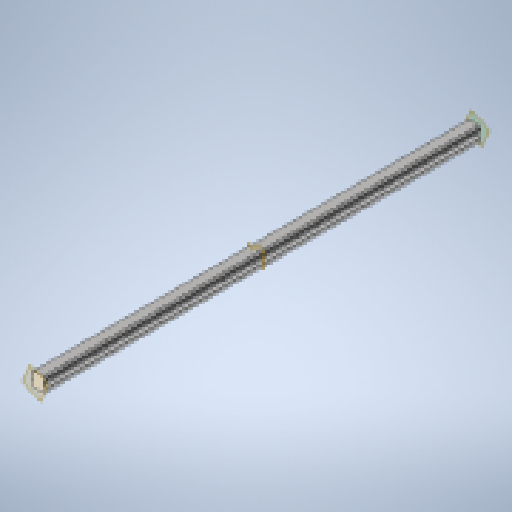
# Autodesk Inventor part: HGR15_Y_RAIL
Saved by Autodesk Inventor 2025.2 (Build 292293000, 293)
## iProperties
Created: 2026-02-05
Part Number: HGR15_Y_RAIL
Material: Generic
Document SubType Name: Modeling
Designer: composite
Density: 1 g/cm^3
Appearance: Default
Author: composite
Autodesk Inventor part; units mm, degrees
ref_plane "YZ Plane" through (0, 0, 0) normal (1, 0, 0) x (0, 1, 0)
ref_plane "XZ Plane" through (0, 0, 0) normal (0, 1, 0) x (-1, 0, 0)
ref_plane "XY Plane" through (0, 0, 0) normal (0, 0, 1) x (1, 0, 0)
derived "HGR15_REPRESENTATIVE.ipt"
sketch "hgr15 REP SKETCH" plane through (-6.8, 0, 100) normal (0, 0, 1) x (1, 0, 0)
  arc A0 (-0.4071, 3.9505) -> (-0.7, 3.2434) centre (0.3, 3.2434) ccw
  line L0 (-0.7, 3.2434) -> (-0.7, 0.7)
  line L1 (-0.7, 0.7) -> (0, 0)
  line L2 (0, 0) -> (13.6, 0)
  line L3 (13.6, 0) -> (14.3, 0.7)
  line L4 (14.3, 0.7) -> (14.3, 3.2434)
  arc A1 (14.3, 3.2434) -> (14.0071, 3.9505) centre (13.3, 3.2434) ccw
  line L5 (14.0071, 3.9505) -> (11.6872, 6.2704)
  arc A2 (11.57, 6.5533) -> (11.6872, 6.2704) centre (11.97, 6.5533) ccw
  line L6 (11.57, 6.5533) -> (11.57, 8.1153)
  arc A3 (11.6872, 8.3982) -> (11.57, 8.1153) centre (11.97, 8.1153) ccw
  line L7 (11.6872, 8.3982) -> (11.8816, 8.5926)
  arc A4 (11.8816, 8.5926) -> (12.0706, 9.0718) centre (11.6914, 8.9445) ccw
  arc A5 (13.2785, 10.4123) -> (12.0706, 9.0718) centre (13.6562, 8.8576) ccw
  arc A6 (13.2785, 10.4123) -> (13.5743, 10.7128) centre (13.1841, 10.801) ccw
  line L8 (13.5743, 10.7128) -> (13.6062, 10.8541)
  arc A7 (13.8606, 11.1421) -> (13.6062, 10.8541) centre (13.9964, 10.7658) ccw
  line L9 (13.8606, 11.1421) -> (14.0357, 11.2052)
  arc A8 (14.0357, 11.2052) -> (14.3, 11.5815) centre (13.9, 11.5815) ccw
  line L10 (14.3, 11.5815) -> (14.3, 12.3375)
  arc A9 (14.3, 12.3375) -> (14.0187, 12.7195) centre (13.9, 12.3375) ccw
  line L11 (14.0187, 12.7195) -> (13.8777, 12.7633)
  arc A10 (13.6053, 13.0612) -> (13.8777, 12.7633) centre (13.9964, 13.1453) ccw
  line L12 (13.6053, 13.0612) -> (13.575, 13.2021)
  arc A11 (13.575, 13.2021) -> (13.2784, 13.5067) centre (13.184, 13.118) ccw
  arc A12 (12.074, 14.8234) -> (13.2784, 13.5067) centre (13.6562, 15.0614) ccw
  arc A13 (12.074, 14.8234) -> (11.8861, 14.9629) centre (11.7521, 14.586) ccw
  line L13 (11.8861, 14.9629) -> (11.849, 15)
  line L14 (11.849, 15) -> (1.751, 15)
  line L15 (1.751, 15) -> (1.7139, 14.9629)
  arc A14 (1.7139, 14.9629) -> (1.526, 14.8234) centre (1.8479, 14.586) ccw
  arc A15 (0.3216, 13.5067) -> (1.526, 14.8234) centre (-0.0562, 15.0614) ccw
  arc A16 (0.3216, 13.5067) -> (0.025, 13.2021) centre (0.416, 13.118) ccw
  line L16 (0.025, 13.2021) -> (-0.0053, 13.0612)
  arc A17 (-0.2777, 12.7633) -> (-0.0053, 13.0612) centre (-0.3964, 13.1453) ccw
  line L17 (-0.2777, 12.7633) -> (-0.4187, 12.7195)
  arc A18 (-0.4187, 12.7195) -> (-0.7, 12.3375) centre (-0.3, 12.3375) ccw
  line L18 (-0.7, 12.3375) -> (-0.7, 11.5815)
  arc A19 (-0.7, 11.5815) -> (-0.4357, 11.2052) centre (-0.3, 11.5815) ccw
  line L19 (-0.4357, 11.2052) -> (-0.2606, 11.1421)
  arc A20 (-0.0062, 10.8541) -> (-0.2606, 11.1421) centre (-0.3964, 10.7658) ccw
  line L20 (-0.0062, 10.8541) -> (0.0257, 10.7128)
  arc A21 (0.0257, 10.7128) -> (0.3215, 10.4123) centre (0.4159, 10.801) ccw
  arc A22 (1.5294, 9.0718) -> (0.3215, 10.4123) centre (-0.0562, 8.8576) ccw
  arc A23 (1.5294, 9.0718) -> (1.7184, 8.5926) centre (1.9086, 8.9445) ccw
  line L21 (1.7184, 8.5926) -> (1.9128, 8.3982)
  arc A24 (2.03, 8.1153) -> (1.9128, 8.3982) centre (1.63, 8.1153) ccw
  line L22 (2.03, 8.1153) -> (2.03, 6.5533)
  arc A25 (1.9128, 6.2704) -> (2.03, 6.5533) centre (1.63, 6.5533) ccw
  line L23 (1.9128, 6.2704) -> (-0.4071, 3.9505)
  point P0 (6.8, 0)
extrude "Extrusion1" add sketch "hgr15 REP SKETCH" along normal blind 5 and the other way blind 5
ref_plane "Work Plane1" through (0, 0.7, 105) normal (1, 0, 0) x (0, 0, -1)
ref_plane "Work Plane2" through (-6.8, 0, 100) normal (0, 0, 1) x (1, 0, 0)
ref_plane "Work Plane3" through (-20, 0, -137.5) normal (0, 0, -1) x (0.4092556, 0.9124198, 0)
ref_plane "Work Plane4" through (13.9751, 75.7463, 337.5) normal (0, 0, 1) x (-0.4092556, -0.9124198, 0)
sketch "Sketch2" plane through (-6.8, 0, 105) normal (0, 0, 1) x (1, 0, 0)
  arc A0 (-0.4071, 3.9505) -> (-0.7, 3.2434) centre (0.3, 3.2434) ccw projected
  line L0 (-0.7, 3.2434) -> (-0.7, 0.7) projected
  line L1 (-0.7, 0.7) -> (0, 0) projected
  line L2 (0, 0) -> (13.6, 0) projected
  line L3 (13.6, 0) -> (14.3, 0.7) projected
  line L4 (14.3, 0.7) -> (14.3, 3.2434) projected
  arc A1 (14.3, 3.2434) -> (14.0071, 3.9505) centre (13.3, 3.2434) ccw projected
  line L5 (14.0071, 3.9505) -> (11.6872, 6.2704) projected
  arc A2 (11.57, 6.5533) -> (11.6872, 6.2704) centre (11.97, 6.5533) ccw projected
  line L6 (11.57, 6.5533) -> (11.57, 8.1153) projected
  arc A3 (11.6872, 8.3982) -> (11.57, 8.1153) centre (11.97, 8.1153) ccw projected
  line L7 (11.6872, 8.3982) -> (11.8816, 8.5926) projected
  arc A4 (11.8816, 8.5926) -> (12.0706, 9.0718) centre (11.6914, 8.9445) ccw projected
  arc A5 (13.2785, 10.4123) -> (12.0706, 9.0718) centre (13.6562, 8.8576) ccw projected
  arc A6 (13.2785, 10.4123) -> (13.5743, 10.7128) centre (13.1841, 10.801) ccw projected
  line L8 (13.5743, 10.7128) -> (13.6062, 10.8541) projected
  arc A7 (13.8606, 11.1421) -> (13.6062, 10.8541) centre (13.9964, 10.7658) ccw projected
  line L9 (13.8606, 11.1421) -> (14.0357, 11.2052) projected
  arc A8 (14.0357, 11.2052) -> (14.3, 11.5815) centre (13.9, 11.5815) ccw projected
  line L10 (14.3, 11.5815) -> (14.3, 12.3375) projected
  arc A9 (14.3, 12.3375) -> (14.0187, 12.7195) centre (13.9, 12.3375) ccw projected
  line L11 (14.0187, 12.7195) -> (13.8777, 12.7633) projected
  arc A10 (13.6053, 13.0612) -> (13.8777, 12.7633) centre (13.9964, 13.1453) ccw projected
  line L12 (13.6053, 13.0612) -> (13.575, 13.2021) projected
  arc A11 (13.575, 13.2021) -> (13.2784, 13.5067) centre (13.184, 13.118) ccw projected
  arc A12 (12.074, 14.8234) -> (13.2784, 13.5067) centre (13.6562, 15.0614) ccw projected
  arc A13 (12.074, 14.8234) -> (11.8861, 14.9629) centre (11.7521, 14.586) ccw projected
  line L13 (11.8861, 14.9629) -> (11.849, 15) projected
  line L14 (11.849, 15) -> (1.751, 15) projected
  line L15 (1.751, 15) -> (1.7139, 14.9629) projected
  arc A14 (1.7139, 14.9629) -> (1.526, 14.8234) centre (1.8479, 14.586) ccw projected
  arc A15 (0.3216, 13.5067) -> (1.526, 14.8234) centre (-0.0562, 15.0614) ccw projected
  arc A16 (0.3216, 13.5067) -> (0.025, 13.2021) centre (0.416, 13.118) ccw projected
  line L16 (0.025, 13.2021) -> (-0.0053, 13.0612) projected
  arc A17 (-0.2777, 12.7633) -> (-0.0053, 13.0612) centre (-0.3964, 13.1453) ccw projected
  line L17 (-0.2777, 12.7633) -> (-0.4187, 12.7195) projected
  arc A18 (-0.4187, 12.7195) -> (-0.7, 12.3375) centre (-0.3, 12.3375) ccw projected
  line L18 (-0.7, 12.3375) -> (-0.7, 11.5815) projected
  arc A19 (-0.7, 11.5815) -> (-0.4357, 11.2052) centre (-0.3, 11.5815) ccw projected
  line L19 (-0.4357, 11.2052) -> (-0.2606, 11.1421) projected
  arc A20 (-0.0062, 10.8541) -> (-0.2606, 11.1421) centre (-0.3964, 10.7658) ccw projected
  line L20 (-0.0062, 10.8541) -> (0.0257, 10.7128) projected
  arc A21 (0.0257, 10.7128) -> (0.3215, 10.4123) centre (0.4159, 10.801) ccw projected
  arc A22 (1.5294, 9.0718) -> (0.3215, 10.4123) centre (-0.0562, 8.8576) ccw projected
  arc A23 (1.5294, 9.0718) -> (1.7184, 8.5926) centre (1.9086, 8.9445) ccw projected
  line L21 (1.7184, 8.5926) -> (1.9128, 8.3982) projected
  arc A24 (2.03, 8.1153) -> (1.9128, 8.3982) centre (1.63, 8.1153) ccw projected
  line L22 (2.03, 8.1153) -> (2.03, 6.5533) projected
  arc A25 (1.9128, 6.2704) -> (2.03, 6.5533) centre (1.63, 6.5533) ccw projected
  line L23 (1.9128, 6.2704) -> (-0.4071, 3.9505) projected
  point P0 (6.8, 0)
extrude "Extrusion2" add sketch "Sketch2" along normal blind 229.5
sketch "Sketch3" plane through (6.8, 0, 95) normal (0, 0, -1) x (-1, 0, 0)
  arc A0 (14.3, 3.2434) -> (14.0071, 3.9505) centre (13.3, 3.2434) ccw projected
  line L0 (14.0071, 3.9505) -> (11.6872, 6.2704) projected
  arc A1 (11.57, 6.5533) -> (11.6872, 6.2704) centre (11.97, 6.5533) ccw projected
  line L1 (11.57, 6.5533) -> (11.57, 8.1153) projected
  arc A2 (11.6872, 8.3982) -> (11.57, 8.1153) centre (11.97, 8.1153) ccw projected
  line L2 (11.6872, 8.3982) -> (11.8816, 8.5926) projected
  arc A3 (11.8816, 8.5926) -> (12.0706, 9.0718) centre (11.6914, 8.9445) ccw projected
  arc A4 (13.2785, 10.4123) -> (12.0706, 9.0718) centre (13.6562, 8.8576) ccw projected
  arc A5 (13.2785, 10.4123) -> (13.5743, 10.7128) centre (13.1841, 10.801) ccw projected
  line L3 (13.5743, 10.7128) -> (13.6062, 10.8541) projected
  arc A6 (13.8606, 11.1421) -> (13.6062, 10.8541) centre (13.9964, 10.7658) ccw projected
  line L4 (13.8606, 11.1421) -> (14.0357, 11.2052) projected
  arc A7 (14.0357, 11.2052) -> (14.3, 11.5815) centre (13.9, 11.5815) ccw projected
  line L5 (14.3, 11.5815) -> (14.3, 12.3375) projected
  arc A8 (14.3, 12.3375) -> (14.0187, 12.7195) centre (13.9, 12.3375) ccw projected
  line L6 (14.0187, 12.7195) -> (13.8777, 12.7633) projected
  arc A9 (13.6053, 13.0612) -> (13.8777, 12.7633) centre (13.9964, 13.1453) ccw projected
  line L7 (13.6053, 13.0612) -> (13.575, 13.2021) projected
  arc A10 (13.575, 13.2021) -> (13.2784, 13.5067) centre (13.184, 13.118) ccw projected
  arc A11 (12.074, 14.8234) -> (13.2784, 13.5067) centre (13.6562, 15.0614) ccw projected
  arc A12 (12.074, 14.8234) -> (11.8861, 14.9629) centre (11.7521, 14.586) ccw projected
  line L8 (11.8861, 14.9629) -> (11.849, 15) projected
  line L9 (11.849, 15) -> (1.751, 15) projected
  line L10 (1.751, 15) -> (1.7139, 14.9629) projected
  arc A13 (1.7139, 14.9629) -> (1.526, 14.8234) centre (1.8479, 14.586) ccw projected
  arc A14 (0.3216, 13.5067) -> (1.526, 14.8234) centre (-0.0562, 15.0614) ccw projected
  arc A15 (0.3216, 13.5067) -> (0.025, 13.2021) centre (0.416, 13.118) ccw projected
  line L11 (0.025, 13.2021) -> (-0.0053, 13.0612) projected
  arc A16 (-0.2777, 12.7633) -> (-0.0053, 13.0612) centre (-0.3964, 13.1453) ccw projected
  line L12 (-0.2777, 12.7633) -> (-0.4187, 12.7195) projected
  arc A17 (-0.4187, 12.7195) -> (-0.7, 12.3375) centre (-0.3, 12.3375) ccw projected
  line L13 (-0.7, 12.3375) -> (-0.7, 11.5815) projected
  arc A18 (-0.7, 11.5815) -> (-0.4357, 11.2052) centre (-0.3, 11.5815) ccw projected
  line L14 (-0.4357, 11.2052) -> (-0.2606, 11.1421) projected
  arc A19 (-0.0062, 10.8541) -> (-0.2606, 11.1421) centre (-0.3964, 10.7658) ccw projected
  line L15 (-0.0062, 10.8541) -> (0.0257, 10.7128) projected
  arc A20 (0.0257, 10.7128) -> (0.3215, 10.4123) centre (0.4159, 10.801) ccw projected
  arc A21 (1.5294, 9.0718) -> (0.3215, 10.4123) centre (-0.0562, 8.8576) ccw projected
  arc A22 (1.5294, 9.0718) -> (1.7184, 8.5926) centre (1.9086, 8.9445) ccw projected
  line L16 (1.7184, 8.5926) -> (1.9128, 8.3982) projected
  arc A23 (2.03, 8.1153) -> (1.9128, 8.3982) centre (1.63, 8.1153) ccw projected
  line L17 (2.03, 8.1153) -> (2.03, 6.5533) projected
  arc A24 (1.9128, 6.2704) -> (2.03, 6.5533) centre (1.63, 6.5533) ccw projected
  line L18 (1.9128, 6.2704) -> (-0.4071, 3.9505) projected
  arc A25 (-0.4071, 3.9505) -> (-0.7, 3.2434) centre (0.3, 3.2434) ccw projected
  line L19 (-0.7, 3.2434) -> (-0.7, 0.7) projected
  line L20 (-0.7, 0.7) -> (0, 0) projected
  line L21 (0, 0) -> (13.6, 0) projected
  line L22 (13.6, 0) -> (14.3, 0.7) projected
  line L23 (14.3, 0.7) -> (14.3, 3.2434) projected
  point P0 (6.8, 0)
extrude "Extrusion3" add sketch "Sketch3" along normal blind 229.5
body "Solid1"
